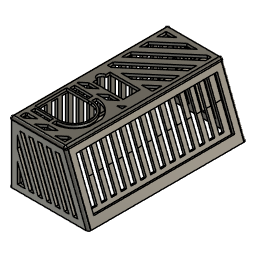
Bearhack Blood Bag Agitator Base (Autodesk Fusion 360 design; units mm, degrees)
part number: 2025-04-05-12-08-34-611
Autodesk Fusion 360 part; units mm, degrees
note: some values were not read from the file. Chosen so that the rebuilt part matches the saved one: which bodies a step acts on; which face or edge a step refers to. Set by a fixed rule: which sketch regions a step uses.
sketch "Sketch1" plane through (0, 0, 0) normal (0, 0, 1) x (1, 0, 0)
  line L0 (0, 0) -> (90, 0)
  line L1 (90, 0) -> (90, 150)
  line L2 (90, 150) -> (0, 150)
  line L3 (0, 150) -> (0, 0)
  constraint horizontal L0
  constraint vertical L1
  constraint horizontal L2
  constraint vertical L3
  constraint coincident L0.start L3.end
extrude "Extrude1" add sketch "Sketch1" along normal blind 70 makes body 1
sketch "Sketch2" plane through (0, 0, 0) normal (0, -1, 0) x (1, 0, 0)
  line L0 (0, 0) -> (90, 0)
  line L1 (90, 0) -> (90, 70)
  line L2 (90, 70) -> (0, 70)
  line L3 (0, 70) -> (0, 0)
  line L4 (90, 0) -> (63.0727, 70)
  constraint coincident L0.end L1.start
  constraint coincident L2 L4.end
extrude "Extrude2" cut sketch "Sketch2" against normal blind 230 contours L1 L2 L4 bodies 1
extrude "Extrude3" add 1 faces at (51.0242, 0, 23.3333) along direction (0, -1, 0) blind 10 on bodies 1 bodies 1
extrude "Extrude4" add 1 faces at (51.0242, -10, 23.3333) along direction (0, -1, 0) blind 20 on bodies 1 bodies 1
shell "Shell1" thickness 3 removed faces 1 at (30, 90, 0) on bodies 1
sketch "Sketch3" plane through (78.3989, 0, 30.1582) normal (0.933327, 0, 0.359028) x (0, 1, 0)
  line L0 (150, -32.3125) -> (150, 42.688)
  line L1 (150, 42.688) -> (-30, 42.688)
  line L2 (-30, 42.688) -> (-30, -32.3125)
  line L3 (-30, -32.3125) -> (150, -32.3125)
sketch "Sketch4" plane through (78.3989, 0, 30.1582) normal (0.933327, 0, 0.359028) x (0, 1, 0)
  line L0 (-30.3562, 42.7788) -> (-20.3562, 42.7788)
  line L1 (-20.3562, 42.7788) -> (-20.3562, -32.6839)
  line L2 (-20.3562, -32.6839) -> (-30.3562, -32.6839)
  line L3 (-30.3562, -32.6839) -> (-30.3562, 42.7788)
  line L4 (-30.3562, 42.7788) -> (149.3651, 42.7788)
  line L5 (149.3651, 42.7788) -> (149.3651, 33.0798)
  line L6 (149.3651, 33.0798) -> (-30.3562, 33.0798)
  line L7 (-30.3562, 33.0798) -> (-30.3562, 42.7788)
  line L8 (-20.3562, 33.0798) -> (140.0853, 33.0798)
  line L9 (140.0853, 33.0798) -> (140.0853, -22.1404)
  line L10 (140.0853, -22.1404) -> (-20.3562, -22.1404)
  line L11 (-20.3562, -22.1404) -> (-20.3562, 33.0798)
  dimension "d10" = 10
  constraint horizontal L0
  constraint vertical L1
  constraint horizontal L2
  constraint vertical L3
  constraint horizontal L4
  constraint vertical L5
  constraint horizontal L6
  constraint vertical L7
  constraint horizontal L8
  constraint vertical L9
  constraint horizontal L10
  constraint vertical L11
  constraint coincident L1 L8.start
  constraint coincident L6 L8.start
  measures "d10" distance of L0.start L0.end
extrude "Extrude5" cut sketch "Sketch4" against normal blind 10 contours L1 L6 L8 L9 L10 L11 bodies 1
fillet "Fillet1" radius 2.5 8 edges at (63.0727, 60, 70) (76.5363, -30, 35) (31.5363, -30, 70) (0, -30, 35) (31.5363, 150, 70) (0, 60, 70) (0, 150, 35) (76.5363, 150, 35) on bodies 1
sketch "Sketch5" plane through (0, 150, 0) normal (0, 1, 0) x (-1, 0, 0)
  line L0 (-2.5, 0) -> (-2.5, 67.5)
  line L1 (-2.5, 67.5) -> (-61.3558, 67.5)
  line L2 (-61.3558, 67.5) -> (-87.3214, 0)
  line L3 (-87.3214, 0) -> (-2.5, 0)
  line L4 (-84.235, 8.0233) -> (-74.1931, 3.5334)
  line L5 (-74.6149, 33.0319) -> (-64.3483, 29.0825)
  line L6 (-76, 0) -> (-64.7528, 29.2382)
  line L7 (-64.3483, 29.0825) -> (-49.57, 67.5)
  line L8 (-49.57, 67.5) -> (-46.57, 67.5)
  line L9 (-76, 0) -> (-73, 0)
  line L10 (-73, 0) -> (-46.57, 67.5)
  line L11 (-64.3483, 29.0825) -> (-76, 0)
  line L12 (-46.57, 67.5) -> (-73, 0)
  line L13 (-76, 0) -> (-49.57, 67.5)
  line L14 (-46.57, 67.5) -> (-73, 0)
  dimension "d15" = 11
  dimension "d16" = 11
  dimension "d17" = 3
  dimension "d18" = 3
  constraint coincident L2 L4.start
  constraint coincident L2 L5.start
  constraint perpendicular L2 L5
  constraint coincident L3 L6.start
  constraint coincident L5 L6.end
  constraint perpendicular L5 L6
  constraint coincident L1 L7.end
  constraint perpendicular L5 L7
  constraint parallel L1 L8
  constraint parallel L3 L9
  measures "d15" distance of L4.start L4.end
  measures "d16" distance of L5.start L5.end
  measures "d17" distance of L7.end L8.end
  measures "d18" distance of L6.start L9.end
extrude "Extrude6" add sketch "Sketch5" against normal blind 177 contours L1 L3 L7 L8 L9 L10 L11 L12 L14 bodies 1
sketch "Sketch6" plane through (0, 0, 70) normal (0, 0, 1) x (-1, 0, 0)
  line L0 (-2.5, -147.5) -> (-2.5, 27.5)
  line L1 (-2.5, 27.5) -> (-61.3558, 27.5)
  line L2 (-61.3558, 27.5) -> (-61.3558, -147.5)
  line L3 (-61.3558, -147.5) -> (-2.5, -147.5)
  line L4 (-34.5239, 27.5) -> (-34.5239, -147.5)
  constraint coincident L1 L4.start
  constraint coincident L3 L4.end
  constraint perpendicular L3 L4
sketch "Sketch7" plane through (0, 0, 70) normal (0, 0, 1) x (-1, 0, 0)
sketch "Sketch8" plane through (0, 0, 70) normal (0, 0, 1) x (-1, 0, 0)
  line L0 (-2.4448, 27.6981) -> (-2.4448, -147.9055)
  line L1 (-2.4448, 27.6981) -> (-61.3695, 27.6981)
  line L2 (-2.4448, 27.6981) -> (-31.8997, 27.6981)
  line L3 (-31.8997, 27.6981) -> (-31.8997, -60.1039)
  line L4 (-31.8997, -60.1039) -> (-2.4448, -60.1039)
  line L5 (-2.4448, -60.1039) -> (-2.4448, 27.6981)
  line L6 (-31.8997, -60.1039) -> (-14.534, -60.1039)
  line L7 (-31.8997, -60.1039) -> (-14.8997, -60.1039)
  line L8 (-14.8997, -60.1039) -> (-14.8997, -50.6039)
  line L9 (-14.8997, -50.6039) -> (-31.8997, -50.6039)
  line L10 (-31.8997, -50.6039) -> (-48.8997, -50.6039)
  line L11 (-48.8997, -50.6039) -> (-48.8997, -69.6039)
  line L12 (-48.8997, -69.6039) -> (-14.8997, -69.6039)
  line L13 (-14.8997, -69.6039) -> (-14.8997, -60.1039)
  dimension "d21" = 87.802
  dimension "d22" = 17
  dimension "d23" = 9.5
  dimension "d24" = 17
  dimension "d25" = 19
  dimension "d26" = 34
  constraint vertical L0
  constraint perpendicular L0 L1
  constraint horizontal L2
  constraint vertical L3
  constraint horizontal L4
  constraint vertical L5
  constraint coincident L4 L6.end
  constraint perpendicular L3 L7
  constraint perpendicular L7 L8
  constraint coincident L3 L9.end
  constraint perpendicular L3 L9
  constraint perpendicular L3 L10
  constraint perpendicular L10 L11
  constraint perpendicular L11 L12
  measures "d21" distance of L0.start L4.end
  measures "d22" distance of L3.end L7.end
  measures "d23" distance of L7.end L8.end
  measures "d24" distance of L9.end L10.end
  measures "d25" distance of L10.end L11.end
  measures "d26" distance of L11.end L12.end
extrude "Extrude7" cut sketch "Sketch8" against normal blind 10 contours L3 L4 L6 L7 L8 L9 | L3 L4 L6 L7 L10 L11 L12 L13 bodies 1
sketch "Sketch9" plane through (65.799, 0, 25.3113) normal (0.933327, 0, 0.359028) x (0, 1, 0)
  line L0 (147, 4.0407) -> (147, 44.6668)
  line L1 (147, 44.6668) -> (-27, 44.6668)
  line L2 (-27, 44.6668) -> (-27, 4.0407)
  line L3 (-27, 4.0407) -> (147, 4.0407)
split "Split1" by plane through (0, -10, 67) normal (0, 0, -1) bodies 1 makes body 2 at (64.9666, 56.868, 20.5167)
split "Split2" by plane through (0, -27, 0) normal (0, 1, 0) bodies 2 makes body 3 at (64.9666, 56.868, 20.5167)
split "Split3" by plane through (90, 147, 0) normal (0, -1, 0) bodies 3 makes body 4 at (3, 31, 22.3333) makes body 5 at (88.7826, 86.6951, 3.1646) makes body 6 at (64.9666, 56.868, 20.5167)
sketch "Sketch10" plane through (65.799, 0, 25.3113) normal (0.933327, 0, 0.359028) x (0, 1, 0)
  line L0 (147, 4.0407) -> (147, 44.6668)
  line L1 (147, 44.6668) -> (-27, 44.6668)
  line L2 (-27, 44.6668) -> (-27, 4.0407)
  line L3 (-27, 4.0407) -> (147, 4.0407)
  line L4 (-22.1835, 40.9094) -> (140.4236, 40.9094)
  line L5 (140.4236, 40.9094) -> (140.4236, -21.9489)
  line L6 (140.4236, -21.9489) -> (-22.1835, -21.9489)
  line L7 (-22.1835, -21.9489) -> (-22.1835, 40.9094)
  line L8 (-15.1763, 40.9094) -> (-15.1763, -21.9489)
  line L9 (-10.024, 40.9094) -> (-10.024, -21.9489)
  line L10 (1.1298, 40.9094) -> (1.1298, -21.9489)
  line L11 (-4.0225, 40.9094) -> (-4.0225, -21.9489)
  line L12 (12.2837, 40.9094) -> (12.2837, -21.9489)
  line L13 (7.1313, 40.9094) -> (7.1313, -21.9489)
  line L14 (23.4375, 40.9094) -> (23.4375, -21.9489)
  line L15 (18.2852, 40.9094) -> (18.2852, -21.9489)
  line L16 (34.5914, 40.9094) -> (34.5914, -21.9489)
  line L17 (29.439, 40.9094) -> (29.439, -21.9489)
  line L18 (45.7452, 40.9094) -> (45.7452, -21.9489)
  line L19 (40.5929, 40.9094) -> (40.5929, -21.9489)
  line L20 (56.899, 40.9094) -> (56.899, -21.9489)
  line L21 (51.7467, 40.9094) -> (51.7467, -21.9489)
  line L22 (68.0529, 40.9094) -> (68.0529, -21.9489)
  line L23 (62.9006, 40.9094) -> (62.9006, -21.9489)
  line L24 (79.2067, 40.9094) -> (79.2067, -21.9489)
  line L25 (74.0544, 40.9094) -> (74.0544, -21.9489)
  line L26 (90.3606, 40.9094) -> (90.3606, -21.9489)
  line L27 (85.2083, 40.9094) -> (85.2083, -21.9489)
  line L28 (101.5144, 40.9094) -> (101.5144, -21.9489)
  line L29 (96.3621, 40.9094) -> (96.3621, -21.9489)
  line L30 (112.6683, 40.9094) -> (112.6683, -21.9489)
  line L31 (107.516, 40.9094) -> (107.516, -21.9489)
  line L32 (123.8221, 40.9094) -> (123.8221, -21.9489)
  line L33 (118.6698, 40.9094) -> (118.6698, -21.9489)
  line L34 (134.976, 40.9094) -> (134.976, -21.9489)
  line L35 (129.8237, 40.9094) -> (129.8237, -21.9489)
  dimension "d31" = 145
  dimension "d32" = 0
  constraint horizontal L4
  constraint vertical L5
  constraint horizontal L6
  constraint vertical L7
  constraint coincident L4 L8.start
  constraint coincident L6 L8.end
  constraint perpendicular L6 L8
  constraint coincident L4 L9.start
  constraint coincident L6 L9.end
  constraint perpendicular L6 L9
extrude "Extrude8" cut sketch "Sketch10" against normal blind 20 contours L3 L5 L6 L34 | L3 L4 L5 L34 | L3 L6 L32 L35 | L3 L4 L32 L35 | L3 L4 L7 L8 | L3 L6 L7 L8 | L3 L6 L30 L33 | L3 L4 L30 L33 | L3 L4 L9 L11 | L3 L6 L9 L11 | L3 L6 L28 L31 | L3 L4 L28 L31 | L3 L4 L10 L13 | L3 L6 L10 L13 | L3 L6 L26 L29 | L3 L4 L26 L29 | L3 L4 L12 L15 | L3 L6 L12 L15 | L3 L6 L24 L27 | L3 L4 L24 L27 | L3 L4 L14 L17 | L3 L6 L14 L17 | L3 L6 L22 L25 | L3 L4 L22 L25 | L3 L4 L16 L19 | L3 L6 L16 L19 | L3 L6 L20 L23 | L3 L4 L20 L23 | L3 L4 L18 L21 | L3 L6 L18 L21 bodies 6
extrude "Extrude9" cut sketch "Sketch10" along normal blind 19 contours L3 L5 L6 L34 | L3 L6 L32 L35 | L3 L6 L7 L8 | L3 L6 L30 L33 | L3 L6 L9 L11 | L3 L6 L28 L31 | L3 L6 L10 L13 | L3 L6 L26 L29 | L3 L6 L12 L15 | L3 L6 L24 L27 | L3 L6 L14 L17 | L3 L6 L22 L25 | L3 L6 L16 L19 | L3 L6 L20 L23 | L3 L6 L18 L21 bodies 6
sketch "Sketch11" plane through (0, 0, 0) normal (-1, 0, 0) x (0, -1, 0)
  line L0 (-147, 67) -> (-147, 0)
  line L1 (-147, 0) -> (27, 0)
  line L2 (27, 0) -> (27, 67)
  line L3 (27, 67) -> (-147, 67)
  line L4 (-141.2186, 62.3564) -> (22.023, 62.3564)
  line L5 (22.023, 62.3564) -> (22.023, 5.6422)
  line L6 (22.023, 5.6422) -> (-141.2186, 5.6422)
  line L7 (-141.2186, 5.6422) -> (-141.2186, 62.3564)
  line L8 (-135.941, 62.3564) -> (-135.941, 5.6422)
  line L9 (-130.6634, 62.3564) -> (-130.6634, 5.6422)
  line L10 (-123.8577, 62.3564) -> (-123.8577, 5.6422)
  line L11 (-118.5801, 62.3564) -> (-118.5801, 5.6422)
  line L12 (-111.7744, 62.3564) -> (-111.7744, 5.6422)
  line L13 (-106.4968, 62.3564) -> (-106.4968, 5.6422)
  line L14 (-99.691, 62.3564) -> (-99.691, 5.6422)
  line L15 (-94.4134, 62.3564) -> (-94.4134, 5.6422)
  line L16 (-87.6077, 62.3564) -> (-87.6077, 5.6422)
  line L17 (-82.3301, 62.3564) -> (-82.3301, 5.6422)
  line L18 (-75.5244, 62.3564) -> (-75.5244, 5.6422)
  line L19 (-70.2468, 62.3564) -> (-70.2468, 5.6422)
  line L20 (-63.441, 62.3564) -> (-63.441, 5.6422)
  line L21 (-58.1634, 62.3564) -> (-58.1634, 5.6422)
  line L22 (-51.3577, 62.3564) -> (-51.3577, 5.6422)
  line L23 (-46.0801, 62.3564) -> (-46.0801, 5.6422)
  line L24 (-39.2744, 62.3564) -> (-39.2744, 5.6422)
  line L25 (-33.9968, 62.3564) -> (-33.9968, 5.6422)
  line L26 (-27.191, 62.3564) -> (-27.191, 5.6422)
  line L27 (-21.9134, 62.3564) -> (-21.9134, 5.6422)
  line L28 (-15.1077, 62.3564) -> (-15.1077, 5.6422)
  line L29 (-9.8301, 62.3564) -> (-9.8301, 5.6422)
  line L30 (-3.0244, 62.3564) -> (-3.0244, 5.6422)
  line L31 (2.2532, 62.3564) -> (2.2532, 5.6422)
  line L32 (9.059, 62.3564) -> (9.059, 5.6422)
  line L33 (14.3366, 62.3564) -> (14.3366, 5.6422)
  dimension "d39" = 145
  dimension "d40" = 0
  constraint horizontal L4
  constraint vertical L5
  constraint horizontal L6
  constraint vertical L7
  constraint coincident L4 L8.start
  constraint coincident L6 L8.end
  constraint perpendicular L6 L8
  constraint coincident L4 L9.start
  constraint coincident L6 L9.end
  constraint perpendicular L6 L9
extrude "Extrude10" cut sketch "Sketch11" against normal blind 25 contours L4 L6 L7 L8 | L4 L6 L9 L10 | L4 L6 L11 L12 | L4 L6 L13 L14 | L4 L6 L15 L16 | L4 L6 L17 L18 | L4 L6 L19 L20 | L4 L6 L21 L22 | L4 L6 L23 L24 | L4 L6 L25 L26 | L4 L6 L27 L28 | L4 L6 L29 L30 | L4 L6 L31 L32 | L4 L5 L6 L33 bodies 4
sketch "Sketch12" plane through (0, 150, 0) normal (0, 1, 0) x (-1, 0, 0)
  line L0 (-2.5, 67) -> (-61.5481, 67)
  line L1 (-61.5481, 67) -> (-87.3214, 0)
  line L2 (-87.3214, 0) -> (-2.5, 0)
  line L3 (-2.5, 0) -> (-2.5, 67)
  line L4 (-57.0167, 60.4018) -> (-77.7137, 6.5982)
  line L5 (-77.7137, 6.5982) -> (-9.0982, 6.5982)
  line L6 (-9.0982, 6.5982) -> (-9.0982, 60.4018)
  line L7 (-9.0982, 60.4018) -> (-57.0167, 60.4018)
  line L8 (-52.0167, 60.4018) -> (-72.7137, 6.5982)
  line L9 (-47.0167, 60.4018) -> (-67.7137, 6.5982)
  line L10 (-42.0167, 60.4018) -> (-62.7137, 6.5982)
  line L11 (-37.0167, 60.4018) -> (-57.7137, 6.5982)
  line L12 (-32.0167, 60.4018) -> (-52.7137, 6.5982)
  line L13 (-27.0167, 60.4018) -> (-47.7137, 6.5982)
  line L14 (-22.0167, 60.4018) -> (-42.7137, 6.5982)
  line L15 (-17.0167, 60.4018) -> (-37.7137, 6.5982)
  line L16 (-12.0167, 60.4018) -> (-32.7137, 6.5982)
  line L17 (-7.0167, 60.4018) -> (-27.7137, 6.5982)
  line L18 (-2.0167, 60.4018) -> (-22.7137, 6.5982)
  line L19 (2.9833, 60.4018) -> (-17.7137, 6.5982)
  dimension "d43" = -6.5982
  dimension "d46" = 60
  dimension "d47" = 0
extrude "Extrude11" cut sketch "Sketch12" against normal blind 1000 contours L5 L6 L17 L18 | L5 L6 L19 | L5 L7 L15 L16 | L5 L7 L13 L14 | L5 L7 L11 L12 | L5 L7 L9 L10 | L4 L5 L7 L8 bodies 2 3
sketch "Sketch13" plane through (0, 0, 70) normal (0, 0, 1) x (-1, 0, 0)
  line L0 (-48.8997, -50.6039) -> (-14.8997, -50.6039)
  line L1 (-14.8997, -50.6039) -> (-14.8997, -69.6039)
  line L2 (-14.8997, -69.6039) -> (-48.8997, -69.6039)
  line L3 (-48.8997, -69.6039) -> (-48.8997, -50.6039)
  line L4 (-2.5, -147.5) -> (-2.5, 27.5)
  line L5 (-2.5, 27.5) -> (-61.3558, 27.5)
  line L6 (-61.3558, 27.5) -> (-61.3558, -147.5)
  line L7 (-61.3558, -147.5) -> (-2.5, -147.5)
  line L8 (-61.3558, -69.6039) -> (-2.5, -69.6039)
  line L9 (-61.3558, -50.1205) -> (-2.5, -50.6039)
  line L10 (-61.3558, -50.1205) -> (-61.3558, 27.5)
  line L11 (-61.3558, 27.5) -> (-2.5, 27.5)
  line L12 (-2.5, -50.6039) -> (-2.5, 27.5)
  line L13 (-2.5, -69.6039) -> (-2.5, -147.5)
  line L14 (-61.3558, -147.5) -> (-2.5, -147.5)
  line L15 (-61.3558, -147.5) -> (-61.3558, -69.6039)
  line L16 (-54.8622, -141.0064) -> (-8.9936, -141.0064)
  line L17 (-8.9936, -76.0974) -> (-8.9936, -141.0064)
  line L18 (-54.8622, -76.0974) -> (-8.9936, -76.0974)
  line L19 (-54.8622, -141.0064) -> (-54.8622, -76.0974)
  line L20 (-54.8618, 21.006) -> (-8.994, 21.006)
  line L21 (-8.994, -44.0563) -> (-8.994, 21.006)
  line L22 (-54.8618, -43.6796) -> (-8.994, -44.0563)
  line L23 (-54.8618, -43.6796) -> (-54.8618, 21.006)
  circle A0 centre (-32.3602, -11.431) radius 32.4399
  circle A1 centre (-32.3602, -11.431) radius 20
  dimension "d50" = 6.4936
  dimension "d51" = -6.494
  dimension "d52" = 40
  constraint coincident L6 L8.start
  constraint coincident L4 L8.end
  constraint perpendicular L4 L8
  constraint coincident L6 L9.start
  constraint coincident L4 L9.end
  constraint coincident L5.end L6.start
  constraint coincident L4.end L5.start
  constraint coincident L4.start L7.end
  constraint coincident L6.end L7.start
  constraint concentric A0 A1
  measures "d52" diameter of A1
sketch "Sketch14" plane through (0, 0, 70) normal (0, 0, 1) x (-1, 0, 0)
  line L0 (-48.8997, -50.6039) -> (-14.8997, -50.6039)
  line L1 (-14.8997, -50.6039) -> (-14.8997, -69.6039)
  line L2 (-14.8997, -69.6039) -> (-48.8997, -69.6039)
  line L3 (-48.8997, -69.6039) -> (-48.8997, -50.6039)
  line L4 (-2.5, -147.5) -> (-2.5, 27.5)
  line L5 (-2.5, 27.5) -> (-61.3558, 27.5)
  line L6 (-61.3558, 27.5) -> (-61.3558, -147.5)
  line L7 (-61.3558, -147.5) -> (-2.5, -147.5)
  line L8 (-56.3558, 22.5) -> (-56.3558, -142.5)
  line L9 (-56.3558, -142.5) -> (-7.5, -142.5)
  line L10 (-7.5, -142.5) -> (-7.5, 22.5)
  line L11 (-7.5, 22.5) -> (-56.3558, 22.5)
  line L12 (-14.8997, -50.6039) -> (-7.3536, -50.6039)
  line L13 (-7.3536, -50.6039) -> (-7.3536, -45.6039)
  line L14 (-7.3536, -45.6039) -> (-14.8997, -45.6039)
  line L15 (-14.8997, -45.6039) -> (-14.8997, -50.6039)
  line L16 (-14.8997, -50.6039) -> (-56.3558, -50.6039)
  line L17 (-56.3558, -50.6039) -> (-56.3558, -45.6039)
  line L18 (-56.3558, -45.6039) -> (-14.8997, -45.6039)
  line L19 (-14.8997, -45.6039) -> (-14.8997, -50.6039)
  line L20 (-14.8997, -69.6039) -> (-58.0159, -69.6039)
  line L21 (-58.0159, -69.6039) -> (-58.0159, -74.6039)
  line L22 (-58.0159, -74.6039) -> (-14.8997, -74.6039)
  line L23 (-14.8997, -74.6039) -> (-14.8997, -69.6039)
  line L24 (-14.8997, -69.6039) -> (-7.5, -69.6039)
  line L25 (-7.5, -69.6039) -> (-7.5, -74.6039)
  line L26 (-7.5, -74.6039) -> (-14.8997, -74.6039)
  line L27 (-14.8997, -74.6039) -> (-14.8997, -69.6039)
  circle A0 centre (-32.3598, -11.5519) radius 34.0547
  circle A1 centre (-32.3598, -11.5519) radius 25
  circle A2 centre (-32.3598, -11.5519) radius 20
  line L28 (-31.9279, 22.5) -> (-32.7917, -45.6039)
  line L29 (-28.39, 22.5) -> (-28.39, -45.6039)
  line L30 (-32.1062, 8.4465) -> (-7.5, 8.1344)
  line L31 (-32.0427, 13.4461) -> (-7.5, 13.1348)
  line L32 (-32.6769, -36.5499) -> (-7.5, -36.8693)
  line L33 (-32.6135, -31.5503) -> (-7.5, -31.5503)
  line L34 (-35.7929, 22.5) -> (-35.6278, -45.6039)
  dimension "d53" = -5
  dimension "d54" = 5
  dimension "d55" = 5
  dimension "d56" = 50
  dimension "d57" = 40
  constraint horizontal L12
  constraint vertical L13
  constraint horizontal L14
  constraint vertical L15
  constraint coincident L0.end L1.start
  constraint horizontal L16
  constraint vertical L17
  constraint horizontal L18
  constraint vertical L19
  constraint coincident L8 L17.end
  constraint horizontal L20
  constraint vertical L21
  constraint horizontal L22
  constraint vertical L23
  constraint coincident L1.end L2.start
  constraint horizontal L24
  constraint vertical L25
  constraint horizontal L26
  constraint vertical L27
  constraint coincident L10 L25.end
  constraint concentric A0 A1
  constraint concentric A1 A2
  constraint midpoint L11 L28.start
  constraint coincident L18 L28.end
  constraint coincident A0 L28.end
  constraint coincident L11 L29.start
  constraint coincident L18 L29.end
  constraint perpendicular L18 L29
  constraint coincident A2 L30.start
  constraint coincident L28 L30.start
  constraint coincident L10 L30.end
  constraint tangent A2 L30
  constraint coincident A1 L31.start
  constraint coincident L28 L31.start
  constraint coincident L10 L31.end
  constraint tangent A1 L31
  constraint parallel L30 L31
  constraint coincident L28 L32.start
  constraint coincident A1 L32.start
  constraint coincident L10 L32.end
  constraint tangent A1 L32
  constraint coincident A2 L33.start
  constraint coincident L28 L33.start
  constraint coincident L10 L33.end
  constraint perpendicular L10 L33
  constraint coincident L11 L34.start
  constraint midpoint L18 L34.end
  measures "d54" distance of L0.end L14.end
  measures "d55" distance of L1.end L22.end
  measures "d56" diameter of A1
  measures "d57" diameter of A2
extrude "Extrude12" cut sketch "Sketch14" against normal blind 3 contours L10 A0 L32 | L8 A1 A2 L34 | L10 A0 A1 L29 L32 L33 | A1 A2 L28 L34 | A1 L29 L33 | A1 A2 L28 L34 | L10 A0 L31 | L10 A0 A1 L29 L30 L31 | A1 L29 L30 bodies 1
sketch "Sketch15" plane through (0, 0, 70) normal (0, 0, 1) x (-1, 0, 0)
  line L0 (-7.5, 8.1344) -> (-28.39, 8.3993)
  line L1 (-28.39, 8.3993) -> (-28.39, 13.3997)
  line L2 (-28.39, 13.3997) -> (-7.5, 13.1348)
  line L3 (-7.5, 13.1348) -> (-7.5, 8.1344)
  line L4 (-7.5, -36.8693) -> (-28.39, -36.6043)
  line L5 (-28.39, -36.6043) -> (-28.39, -31.5503)
  line L6 (-28.39, -31.5503) -> (-7.5, -31.5503)
  line L7 (-7.5, -31.5503) -> (-7.5, -36.8693)
  arc A0 (-32.0427, 13.4461) -> (-56.3558, -4.5382) centre (-32.3598, -11.5519) ccw
  line L8 (-32.0427, 13.4461) -> (-32.1062, 8.4465)
  arc A1 (-32.1062, 8.4465) -> (-32.6135, -31.5503) centre (-32.3598, -11.5519) ccw
  line L9 (-32.6135, -31.5503) -> (-32.6769, -36.5499)
  arc A2 (-56.3558, -18.5657) -> (-32.6769, -36.5499) centre (-32.3598, -11.5519) ccw
  line L10 (-56.3558, -18.5657) -> (-56.3558, -4.5382)
  line L11 (-48.8997, -50.6039) -> (-14.8997, -50.6039)
  line L12 (-14.8997, -50.6039) -> (-14.8997, -69.6039)
  line L13 (-14.8997, -69.6039) -> (-48.8997, -69.6039)
  line L14 (-48.8997, -69.6039) -> (-48.8997, -50.6039)
  line L15 (-2.5, -147.5) -> (-2.5, 27.5)
  line L16 (-2.5, 27.5) -> (-61.3558, 27.5)
  line L17 (-61.3558, 27.5) -> (-61.3558, -147.5)
  line L18 (-61.3558, -147.5) -> (-2.5, -147.5)
  line L19 (-30.39, 15.4253) -> (-5.5, 15.1096)
  line L20 (-5.5, 15.1096) -> (-5.5, 6.1088)
  line L21 (-5.5, 6.1088) -> (-30.39, 6.4245)
  line L22 (-30.39, 6.4245) -> (-30.39, 15.4253)
  arc A3 (-58.3558, -18.8464) -> (-30.7015, -38.501) centre (-32.3598, -11.5519) ccw
  line L23 (-30.5868, -29.4644) -> (-30.7015, -38.501)
  arc A4 (-30.1331, 6.3098) -> (-30.5868, -29.4644) centre (-32.3598, -11.5519) ccw
  line L24 (-30.0185, 15.3464) -> (-30.1331, 6.3098)
  arc A5 (-30.0185, 15.3464) -> (-58.3558, -4.2575) centre (-32.3598, -11.5519) ccw
  line L25 (-58.3558, -18.8464) -> (-58.3558, -4.2575)
  line L26 (-5.5, -38.8948) -> (-30.39, -38.5791)
  line L27 (-30.39, -38.5791) -> (-30.39, -29.5503)
  line L28 (-30.39, -29.5503) -> (-5.5, -29.5503)
  line L29 (-5.5, -29.5503) -> (-5.5, -38.8948)
  line L30 (-5.5, 6.1088) -> (-5.5, -29.5503)
  line L31 (-5.5, -38.8948) -> (-56.0171, -38.254)
  line L32 (-5.5, 15.1096) -> (-50.2271, 15.6769)
  line L33 (-22.7968, -29.4644) -> (-40, -29.4644)
  line L34 (-25.8858, 6.3098) -> (-35.0575, 6.4837)
  dimension "d60" = -2
  dimension "d61" = -2
  dimension "d62" = -2
  constraint parallel L26 L31
  constraint perpendicular L27 L33
extrude "Extrude13" cut sketch "Sketch15" against normal blind 3 contours L21 A3 L23 A4 L24 L27 L28 L30 L31 L33 L34 bodies 1
extrude "Extrude14" add 1 faces at (31.1608, 38.5693, 69) along direction (-0.012683, -0.99992, 0) blind 0.3 on bodies 1 bodies 1
extrude "Extrude15" add 1 faces at (30.39, 35.3695, 69) along direction (1, 0, 0) blind 0.8 on bodies 1 bodies 1
sketch "Sketch16" plane through (0, 0, 70) normal (0, 0, 1) x (-1, 0, 0)
  line L0 (-30.5879, -29.5503) -> (-30.5868, -29.4644)
  line L1 (-30.5868, -29.4644) -> (-34.1328, -29.4644)
  arc A0 (-32.8396, 6.4417) -> (-34.1328, -29.4644) centre (-32.3598, -11.5519) ccw
  line L2 (-32.8396, 6.4417) -> (-31.1982, 6.4106)
  arc A1 (-30.1331, 6.3098) -> (-31.1982, 6.4106) centre (-32.3598, -11.5519) ccw
  line L3 (-30.1331, 6.3098) -> (-30.1317, 6.4213)
  line L4 (-30.1317, 6.4213) -> (-5.5, 6.1088)
  line L5 (-5.5, 6.1088) -> (-5.5, -29.5503)
  line L6 (-5.5, -29.5503) -> (-30.5879, -29.5503)
  line L7 (-2.5, -147.5) -> (-2.5, 27.5)
  line L8 (-2.5, 27.5) -> (-61.3558, 27.5)
  line L9 (-61.3558, 27.5) -> (-61.3558, -147.5)
  line L10 (-61.3558, -147.5) -> (-2.5, -147.5)
  line L11 (-48.8997, -50.6039) -> (-14.8997, -50.6039)
  line L12 (-14.8997, -50.6039) -> (-14.8997, -69.6039)
  line L13 (-14.8997, -69.6039) -> (-48.8997, -69.6039)
  line L14 (-48.8997, -69.6039) -> (-48.8997, -50.6039)
  arc A2 (-32.0427, 13.4461) -> (-56.3558, -4.5382) centre (-32.3598, -11.5519) ccw
  line L15 (-32.0427, 13.4461) -> (-32.1062, 8.4465)
  arc A3 (-32.1062, 8.4465) -> (-32.6135, -31.5503) centre (-32.3598, -11.5519) ccw
  line L16 (-32.6135, -31.5503) -> (-32.6769, -36.5499)
  arc A4 (-56.3558, -18.5657) -> (-32.6769, -36.5499) centre (-32.3598, -11.5519) ccw
  line L17 (-56.3558, -18.5657) -> (-56.3558, -4.5382)
  line L18 (-7.5, -36.8693) -> (-28.39, -36.6043)
  line L19 (-28.39, -36.6043) -> (-28.39, -31.5503)
  line L20 (-28.39, -31.5503) -> (-7.5, -31.5503)
  line L21 (-7.5, -31.5503) -> (-7.5, -36.8693)
  line L22 (-7.5, 8.1344) -> (-28.39, 8.3993)
  line L23 (-28.39, 8.3993) -> (-28.39, 13.3997)
  line L24 (-28.39, 13.3997) -> (-7.5, 13.1348)
  line L25 (-7.5, 13.1348) -> (-7.5, 8.1344)
  line L26 (-6.5566, 24.3381) -> (-57.6657, 24.3381)
  line L27 (-57.6657, 24.3381) -> (-57.6657, 17.3231)
  line L28 (-57.6657, 17.3231) -> (-6.5566, 17.3231)
  line L29 (-6.5566, 17.3231) -> (-6.5566, 24.3381)
  line L30 (-6.5566, -40.6006) -> (-57.6657, -40.6006)
  line L31 (-57.6657, -40.6006) -> (-57.6657, -47.2147)
  line L32 (-57.6657, -47.2147) -> (-6.5566, -47.2147)
  line L33 (-6.5566, -47.2147) -> (-6.5566, -40.6006)
  line L34 (-6.5566, -75.1124) -> (-57.6657, -75.1124)
  line L35 (-57.6657, -75.1124) -> (-57.6657, -141.8714)
  line L36 (-57.6657, -141.8714) -> (-6.5566, -141.8714)
  line L37 (-6.5566, -141.8714) -> (-6.5566, -75.1124)
  line L38 (21.663, -137.3674) -> (-70.8618, -216.9297)
  line L39 (21.663, -127.3674) -> (-70.8618, -206.9297)
  line L40 (21.663, -117.3674) -> (-70.8618, -196.9297)
  line L41 (21.663, -107.3674) -> (-70.8618, -186.9297)
  line L42 (21.663, -97.3674) -> (-70.8618, -176.9297)
  line L43 (21.663, -87.3674) -> (-70.8618, -166.9297)
  line L44 (21.663, -77.3674) -> (-70.8618, -156.9297)
  line L45 (21.663, -67.3674) -> (-70.8618, -146.9297)
  line L46 (21.663, -57.3674) -> (-70.8618, -136.9297)
  line L47 (21.663, -47.3674) -> (-70.8618, -126.9297)
  line L48 (21.663, -37.3674) -> (-70.8618, -116.9297)
  line L49 (21.663, -27.3674) -> (-70.8618, -106.9297)
  line L50 (21.663, -17.3674) -> (-70.8618, -96.9297)
  line L51 (21.663, -7.3674) -> (-70.8618, -86.9297)
  line L52 (21.663, 2.6326) -> (-70.8618, -76.9297)
  line L53 (21.663, 12.6326) -> (-70.8618, -66.9297)
  line L54 (21.663, 22.6326) -> (-70.8618, -56.9297)
  line L55 (21.663, 32.6326) -> (-70.8618, -46.9297)
  line L56 (21.663, 42.6326) -> (-70.8618, -36.9297)
  line L57 (21.663, 52.6326) -> (-70.8618, -26.9297)
  line L58 (21.663, 62.6326) -> (-70.8618, -16.9297)
  line L59 (21.663, 72.6326) -> (-70.8618, -6.9297)
  line L60 (21.663, 82.6326) -> (-70.8618, 3.0703)
  dimension "d71" = 0
  dimension "d72" = 220
  constraint horizontal L26
  constraint vertical L27
  constraint horizontal L28
  constraint vertical L29
  constraint horizontal L30
  constraint vertical L31
  constraint horizontal L32
  constraint vertical L33
  constraint horizontal L34
  constraint vertical L35
  constraint horizontal L36
  constraint vertical L37
extrude "Extrude16" cut sketch "Sketch16" against normal blind 300 contours L30 L32 L52 L53 | L30 L31 L54 | L30 L32 L33 L50 L51 | L26 L28 L29 L56 L57 | L34 L35 L50 L51 | L34 L35 L37 L46 L47 | L34 L35 L48 L49 | L26 L28 L58 L59 | L35 L36 L37 L44 L45 | L26 L27 L28 L60 | L36 L37 L42 L43 | L36 L37 L40 L41 bodies 1
sketch "Sketch17" plane through (0, 0, 70) normal (0, 0, 1) x (-1, 0, 0)
  line L0 (-57.6657, -135.5824) -> (-6.5566, -91.6335)
  line L1 (-6.5566, -91.6335) -> (-6.5566, -101.6335)
  line L2 (-6.5566, -101.6335) -> (-53.3501, -141.8714)
  line L3 (-53.3501, -141.8714) -> (-57.6657, -141.8714)
  line L4 (-57.6657, -141.8714) -> (-57.6657, -135.5824)
  line L5 (-57.6657, -45.5824) -> (-57.6657, -40.6006)
  line L6 (-57.6657, -40.6006) -> (-51.8722, -40.6006)
  line L7 (-51.8722, -40.6006) -> (-57.6657, -45.5824)
  line L8 (-42.6576, 17.3231) -> (-34.4997, 24.3381)
  line L9 (-34.4997, 24.3381) -> (-22.8705, 24.3381)
  line L10 (-22.8705, 24.3381) -> (-31.0284, 17.3231)
  line L11 (-31.0284, 17.3231) -> (-42.6576, 17.3231)
  line L12 (-11.2413, 24.3381) -> (-6.5566, 24.3381)
  line L13 (-6.5566, 24.3381) -> (-6.5566, 18.3665)
  line L14 (-6.5566, 18.3665) -> (-7.77, 17.3231)
  line L15 (-7.77, 17.3231) -> (-19.3992, 17.3231)
  line L16 (-19.3992, 17.3231) -> (-11.2413, 24.3381)
  line L17 (-57.6657, -75.5824) -> (-57.1191, -75.1124)
  line L18 (-57.1191, -75.1124) -> (-45.4899, -75.1124)
  line L19 (-45.4899, -75.1124) -> (-57.6657, -85.5824)
  line L20 (-57.6657, -85.5824) -> (-57.6657, -75.5824)
  line L21 (-41.7209, -141.8714) -> (-6.5566, -111.6335)
  line L22 (-6.5566, -111.6335) -> (-6.5566, -121.6335)
  line L23 (-6.5566, -121.6335) -> (-30.0917, -141.8714)
  line L24 (-30.0917, -141.8714) -> (-41.7209, -141.8714)
  line L25 (-10.6022, -75.1124) -> (-6.5566, -75.1124)
  line L26 (-6.5566, -75.1124) -> (-6.5566, -81.6335)
  line L27 (-6.5566, -81.6335) -> (-57.6657, -125.5824)
  line L28 (-57.6657, -125.5824) -> (-57.6657, -115.5824)
  line L29 (-57.6657, -115.5824) -> (-10.6022, -75.1124)
  line L30 (-47.9347, -47.2147) -> (-40.243, -40.6006)
  line L31 (-40.243, -40.6006) -> (-28.6138, -40.6006)
  line L32 (-28.6138, -40.6006) -> (-36.3055, -47.2147)
  line L33 (-36.3055, -47.2147) -> (-47.9347, -47.2147)
  line L34 (-57.6657, 17.3231) -> (-57.6657, 24.3381)
  line L35 (-57.6657, 24.3381) -> (-46.1289, 24.3381)
  line L36 (-46.1289, 24.3381) -> (-54.2868, 17.3231)
  line L37 (-54.2868, 17.3231) -> (-57.6657, 17.3231)
  line L38 (-16.9846, -40.6006) -> (-6.5566, -40.6006)
  line L39 (-6.5566, -40.6006) -> (-6.5566, -41.6335)
  line L40 (-6.5566, -41.6335) -> (-13.0471, -47.2147)
  line L41 (-13.0471, -47.2147) -> (-24.6763, -47.2147)
  line L42 (-24.6763, -47.2147) -> (-16.9846, -40.6006)
  line L43 (-57.6657, -95.5824) -> (-33.8607, -75.1124)
  line L44 (-33.8607, -75.1124) -> (-22.2315, -75.1124)
  line L45 (-22.2315, -75.1124) -> (-57.6657, -105.5824)
  line L46 (-57.6657, -105.5824) -> (-57.6657, -95.5824)
  line L47 (-18.4625, -141.8714) -> (-6.5566, -131.6335)
  line L48 (-6.5566, -131.6335) -> (-6.5566, -141.6335)
  line L49 (-6.5566, -141.6335) -> (-6.8333, -141.8714)
  line L50 (-6.8333, -141.8714) -> (-18.4625, -141.8714)
  line L51 (-30.5879, -29.5503) -> (-30.5868, -29.4644)
  line L52 (-30.5868, -29.4644) -> (-34.1328, -29.4644)
  arc A0 (-32.8396, 6.4417) -> (-34.1328, -29.4644) centre (-32.3598, -11.5519) ccw
  line L53 (-32.8396, 6.4417) -> (-31.1982, 6.4106)
  arc A1 (-30.1331, 6.3098) -> (-31.1982, 6.4106) centre (-32.3598, -11.5519) ccw
  line L54 (-30.1331, 6.3098) -> (-30.1317, 6.4213)
  line L55 (-30.1317, 6.4213) -> (-5.5, 6.1088)
  line L56 (-5.5, 6.1088) -> (-5.5, -29.5503)
  line L57 (-5.5, -29.5503) -> (-30.5879, -29.5503)
  line L58 (-2.5, -147.5) -> (-2.5, 27.5)
  line L59 (-2.5, 27.5) -> (-61.3558, 27.5)
  line L60 (-61.3558, 27.5) -> (-61.3558, -147.5)
  line L61 (-61.3558, -147.5) -> (-2.5, -147.5)
  line L62 (-48.8997, -50.6039) -> (-14.8997, -50.6039)
  line L63 (-14.8997, -50.6039) -> (-14.8997, -69.6039)
  line L64 (-14.8997, -69.6039) -> (-48.8997, -69.6039)
  line L65 (-48.8997, -69.6039) -> (-48.8997, -50.6039)
  arc A2 (-32.0427, 13.4461) -> (-56.3558, -4.5382) centre (-32.3598, -11.5519) ccw
  line L66 (-32.0427, 13.4461) -> (-32.1062, 8.4465)
  arc A3 (-32.1062, 8.4465) -> (-32.6135, -31.5503) centre (-32.3598, -11.5519) ccw
  line L67 (-32.6135, -31.5503) -> (-32.6769, -36.5499)
  arc A4 (-56.3558, -18.5657) -> (-32.6769, -36.5499) centre (-32.3598, -11.5519) ccw
  line L68 (-56.3558, -18.5657) -> (-56.3558, -4.5382)
  line L69 (-7.5, -36.8693) -> (-28.39, -36.6043)
  line L70 (-28.39, -36.6043) -> (-28.39, -31.5503)
  line L71 (-28.39, -31.5503) -> (-7.5, -31.5503)
  line L72 (-7.5, -31.5503) -> (-7.5, -36.8693)
  line L73 (-7.5, 8.1344) -> (-28.39, 8.3993)
  line L74 (-28.39, 8.3993) -> (-28.39, 13.3997)
  line L75 (-28.39, 13.3997) -> (-7.5, 13.1348)
  line L76 (-7.5, 13.1348) -> (-7.5, 8.1344)
  circle A5 centre (-14.8997, -60.1039) radius 4.9008
  constraint midpoint L63 A5.centre
extrude "Extrude17" cut sketch "Sketch17" against normal blind 3 contours L63 A5 picked at (-11.975, -59.6436) bodies 1
move_face "OffsetFaces1" offset -0.2 1 faces at (37.5664, 69.6039, 68) on bodies 1
move_face "OffsetFaces2" offset -0.2 1 faces at (26.2331, 50.6039, 69) on bodies 1
move_face "OffsetFaces3" offset -0.2 2 faces at (14.8997, 53.6033, 69) (14.8997, 66.6044, 68) on bodies 1
move_face "OffsetFaces4" offset -0.2 1 faces at (48.8997, 56.8705, 69) on bodies 1
named bodies: "Top", "Left", "Right", "Back", "Front", "BackWall"
